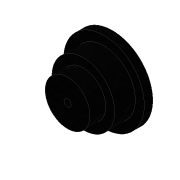
# Autodesk Inventor part: M17 - Coil Support Part
Saved by Autodesk Inventor 2016 (Build 200138000, 138)
## iProperties
Created: 2017-02-27
Part Number: M17 - Coil Support Part
Material: UHMW, Black
Document SubType Name: Modeling
Designer: Fernando
Stock Number: 0
Mass: 152.884 g
Surface Area: 258.005 cm^2
Volume: 162.643 cm^3
Density: 0.94 g/cm^3
Appearance: Black
SurfaceArea_m2: .03
Author: Fernando
Autodesk Inventor part; units mm, degrees
ref_plane "YZ Plane" through (0, 0, 0) normal (1, 0, 0) x (0, 1, 0)
ref_plane "XZ Plane" through (0, 0, 0) normal (0, 1, 0) x (-1, 0, 0)
ref_plane "XY Plane" through (0, 0, 0) normal (0, 0, 1) x (1, 0, 0)
sketch "Sketch2" plane through (0, 0, 0) normal (0, 0, 1) x (1, 0, 0)
  line L0 (-4, 0) -> (-25, 0)
  line L1 (-25, 0) -> (-25, 17.5)
  line L2 (-25, 17.5) -> (-35, 17.5)
  line L3 (-4, 35) -> (-4, 0)
  line L4 (0, 0) -> (0, 29) construction
  line L5 (-4, 35) -> (-19, 35)
  line L6 (-19, 35) -> (-19, 50)
  line L7 (-35, 17.5) -> (-35, 40.5)
  line L8 (-19, 50) -> (-45, 50)
  line L9 (-45, 50) -> (-45, 40.5)
  line L10 (-45, 40.5) -> (-35, 40.5)
  dimension "d11" = 8
  dimension "d13" = 50
  dimension "d28" = 17.5
  dimension "d29" = 35
  dimension "d30" = 15
  dimension "d34" = 70
  dimension "d35" = 50
  dimension "d36" = 23
  dimension "d37" = 90
  constraints: 22 end point, 4 perpendicular, 3 horizontal, 2 vertical, 1 horizontal alignment
  measures "d11" diameter of L3 L4
  measures "d13" diameter of L1 L4
  measures "d28" distance of L0.end L1.end
  measures "d29" distance of L3.start L0.start
  measures "d30" distance between parallel lines of L3 L6
  measures "d34" diameter of L7 L4
  measures "d35" distance between parallel lines of L0 L8
  measures "d36" distance of L2.end L7.end
  measures "d37" diameter of L9 L4
revolve "Revolution1" add sketch "Sketch2" angle 360 about axis through (0, 0, 0) along (0, 1, 0)
chamfer "Chamfer1" distance 5 angle 45 1 edges at (19, 50, 0)
sketch "Sketch3" plane through (0, 50, 0) normal (0, 1, 0) x (1, 0, 0)
  point P0 (0, 0)
  point P1 (0, 35)
  dimension "d38" = 35
  constraints: 1 vertical alignment
  measures "d38" distance of point (0, 35) point (0, 0)
hole "Hole1" at (0, 50, -35) direction (0, -1, 0) diameter 3.242 depth 8 tip angle 118 thread size "M4x0.7" class "6H" standard "ISO Metric profile"
pattern_circular "Circular Pattern1" count 4 over 360 about axis through (0, 42.5, 0) along (0, 1, 0) of "Hole1"
body "Solid2"
